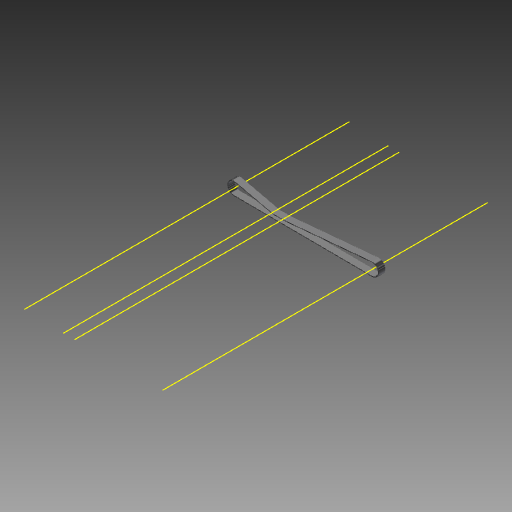
# Autodesk Inventor part: Zahnriemen
Saved by Autodesk Inventor 2019.1 (Build 231200000, 200)
## iProperties
Created: 2018-10-30
Part Number: Zahnriemen
Material: Rubber
Document SubType Name: Modeling
Designer: JochenAlt
Density: 1 g/cm^3
Appearance: Rubber - Black - Version 1.1
CustomPartVersion: 1
Author: JochenAlt
Autodesk Inventor part; units mm, degrees
sketch "Skizzenpfad" plane through (0, 0, 0) normal (0, 0, 1) x (1, 0, 0)
  arc A0 (114.343934, -5.570303) -> (113.874605, 5.547406) centre (114.380472, 0) ccw
  arc A1 (-8.729894, 6.240184) -> (-10.033775, -4.754459) centre (-9.997237, 0.815845) ccw
  arc A2 (24.703327, -1.571154) -> (24.994596, -1.605239) centre (24.999094, -0.305247) ccw
  arc A3 (34.994536, -1.639838) -> (35.117091, -1.634474) centre (34.999034, -0.339846) ccw
  line L0 (35.117091, -1.634474) -> (113.874605, 5.547406)
  line L1 (114.343934, -5.570303) -> (-10.033775, -4.754459)
  line L2 (-8.729894, 6.240184) -> (24.703327, -1.571154)
  line L3 (24.994596, -1.605239) -> (34.994536, -1.639838)
  constraints: 8 end point, 8 point on circle, 4 centre point
ref_plane "Querschnittsebene" through (113.874605, 5.547406, 0) normal (-0.995868, -0.090813, 0) x (0, 0, 1)
ref_plane "Arbeitsebene2" through (114.380472, 0, 0) normal (-1, 0, 0) x (0, 0, 1)
ref_plane "Arbeitsebene3" through (-9.997237, 0.815845, 0) normal (0.99382, -0.1110038, 0) x (0, 0, 1)
sketch "Querschnitt" plane through (113.874605, 5.547406, 0) normal (-0.995868, -0.090813, 0) x (0, 0, 1)
  line L0 (-3, 0.3) -> (3, 0.3)
  line L1 (3, 0.3) -> (3, -0.3)
  line L2 (3, -0.3) -> (-3, -0.3)
  line L3 (-3, -0.3) -> (-3, 0.3)
  line L4 (-3, 0) -> (3, 0) construction
  point P0 (0, 0)
  point P1 (0, 0)
  dimension "d0" = 6
  dimension "d4" = 0.3
  dimension "d5" = 0.3
  constraints: 10 end point, 3 midpoint, 2 parallel, 1 coincident, 1 horizontal, 1 perpendicular, 1 other
  measures "d0" distance between parallel lines of L1 L3
  measures "d4" distance between parallel lines of L2 L4
  measures "d5" distance between parallel lines of L4 L0
sweep "Riemen" add profiles "Querschnitt" path "Skizzenpfad"
equation "\"d0\" = da_B"
equation "\"d4\" = da_a"
equation "\"d5\" = da_a2"
equation "\"da_B\" = 6"
equation "\"da_pb\" = 2.5"
equation "\"da_L\" = 285"
equation "\"da_a\" = 0.3"
equation "\"da_S\" = 1.5"
equation "\"da_Beta\" = 20deg"
equation "\"da_Ht\" = 0.7"
equation "\"da_H\" = 1.3"
equation "\"da_a2\" = 0.3"
body "Solid1"
